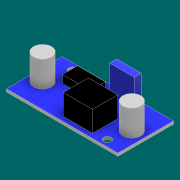
# Autodesk Inventor part: VoltageRegulator
Saved by Autodesk Inventor 2017.3 (Build 213257000, 257)
## iProperties
Created: 2019-12-12
Part Number: VoltageRegulator
Material: Generic
Document SubType Name: Modeling
Designer: Santiago
Density: 1 g/cm^3
Appearance: Default
Author: Santiago
Autodesk Inventor part; units mm, degrees
ref_plane "YZ Plane" through (0, 0, 0) normal (1, 0, 0) x (0, 1, 0)
ref_plane "XZ Plane" through (0, 0, 0) normal (0, 1, 0) x (-1, 0, 0)
ref_plane "XY Plane" through (0, 0, 0) normal (0, 0, 1) x (1, 0, 0)
sketch "Sketch1" plane through (0, 0, 0) normal (0, 0, 1) x (1, 0, 0)
  line L0 (0, 0) -> (43, 0)
  line L1 (43, 0) -> (43, 21.5)
  line L2 (43, 21.5) -> (0, 21.5)
  line L3 (0, 21.5) -> (0, 0)
  dimension "d0" = 43
  dimension "d1" = 21.5
  dimension "d2" = 43
  constraints: 8 end point, 2 perpendicular, 1 horizontal
  measures "d0" distance of L0.start L0.end
  measures "d1" distance of L0.end L1.end
  measures "d2" distance of L1.end L2.end
extrude "Extrusion1" add sketch "Sketch1" along normal blind 1.1
sketch "Sketch2" plane through (0, 0, 1.1) normal (0, 0, 1) x (1, 0, 0)
  line L0 (43, 21.5) -> (0, 21.5) projected
  line L1 (0, 21.5) -> (6.5, 21.5)
  line L2 (6.5, 21.5) -> (6.5, 19)
  circle A0 centre (6.5, 19) radius 1.5
  line L3 (0, 0) -> (43, 0) projected
  line L4 (43, 0) -> (36.5, 0)
  line L5 (36.5, 0) -> (36.5, 2.5)
  circle A1 centre (36.5, 2.5) radius 1.5
  dimension "d5" = 6.5
  dimension "d6" = 2.5
  dimension "d7" = 3
  dimension "d8" = 6.5
  dimension "d9" = 2.5
  dimension "d10" = 3
  constraints: 8 end point, 2 centre point, 2 coincident, 2 perpendicular, 2 point on line
  measures "d5" distance of L0.end L1.end
  measures "d6" distance of L1.end L2.end
  measures "d7" diameter of A0
  measures "d8" distance of L3.end L4.end
  measures "d9" distance of L4.end L5.end
  measures "d10" diameter of A1
extrude "Extrusion2" cut sketch "Sketch2" against normal blind 1.1
sketch "Sketch3" plane through (0, 0, 1.1) normal (0, 0, 1) x (1, 0, 0)
  circle A0 centre (4.6207, 9.3261) radius 3.5
  circle A1 centre (38.2496, 10.1463) radius 3.5
  point P0 (0, 0)
  dimension "d13" = 7
  dimension "d14" = 7
  constraints: 2 centre point
  measures "d13" diameter of A0
  measures "d14" diameter of A1
extrude "Extrusion3" add sketch "Sketch3" along normal blind 10
sketch "Sketch4" plane through (0, 0, 1.1) normal (0, 0, 1) x (1, 0, 0)
  line L0 (31.8145, 20.2348) -> (31.8145, 17.4683)
  line L1 (31.8145, 17.4683) -> (22.3294, 17.4683)
  line L2 (22.3294, 17.4683) -> (22.3294, 20.2348)
  line L3 (22.3294, 20.2348) -> (31.8145, 20.2348)
  point P0 (0, 0)
  constraints: 8 end point, 3 perpendicular, 1 vertical
extrude "Extrusion4" add sketch "Sketch4" along normal blind 11
sketch "Sketch5" plane through (0, 0, 1.1) normal (0, 0, 1) x (1, 0, 0)
  line L0 (31.4983, 11.4611) -> (31.4983, 1.7389)
  line L1 (31.4983, 1.7389) -> (20.1953, 1.7389)
  line L2 (20.1953, 1.7389) -> (20.1953, 11.4611)
  line L3 (20.1953, 11.4611) -> (31.4983, 11.4611)
  point P0 (0, 0)
  constraints: 8 end point, 3 perpendicular, 1 vertical
extrude "Extrusion5" add sketch "Sketch5" along normal blind 8
sketch "Sketch6" plane through (0, 0, 1.1) normal (0, 0, 1) x (1, 0, 0)
  line L0 (9.0495, 18.4071) -> (19.8493, 18.4071)
  line L1 (19.8493, 18.4071) -> (19.8493, 12.5444)
  line L2 (19.8493, 12.5444) -> (9.0495, 12.5444)
  line L3 (9.0495, 12.5444) -> (9.0495, 18.4071)
  point P0 (0, 0)
  constraints: 8 end point, 3 perpendicular, 1 horizontal
extrude "Extrusion6" add sketch "Sketch6" along normal blind 3
body "Solid1"
